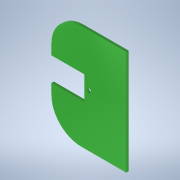
# Autodesk Inventor part: PCB-main
Saved by Autodesk Inventor 2022 (Build 260153000, 153)
## iProperties
Created: 2024-06-04
Part Number: PCB-main
Material: 一般
Document SubType Name: Modeling
Designer: yamashita1
Density: 1 g/cm^3
Appearance: 滑らか - 濃い深緑
Author: yamashita1
Autodesk Inventor part; units mm, degrees
ref_plane "YZ Plane" through (0, 0, 0) normal (1, 0, 0) x (0, 1, 0)
ref_plane "XZ Plane" through (0, 0, 0) normal (0, 1, 0) x (-1, 0, 0)
ref_plane "XY Plane" through (0, 0, 0) normal (0, 0, 1) x (1, 0, 0)
sketch "スケッチ1" plane through (0, 0, 0) normal (0, 0, 1) x (1, 0, 0)
  line L0 (-25, 35) -> (25, 35)
  line L1 (25, 35) -> (25, -35)
  line L2 (25, -35) -> (-25, -35)
  line L3 (-25, -35) -> (-25, 35)
  point P0 (0, 0)
  point P1 (-25, 0)
  point P2 (0, 35)
  dimension "d0" = 50
  dimension "d1" = 70
  constraints: 8 end point, 2 midpoint, 2 parallel, 1 horizontal, 1 horizontal alignment, 1 perpendicular, 1 vertical alignment
  measures "d0" distance of L1.end L2.end
  measures "d1" distance of L0.end L1.end
extrude "押し出し1" add sketch "スケッチ1" along normal blind 1.6
sketch "スケッチ2" plane through (0, 0, 1.6) normal (0, 0, 1) x (1, 0, 0)
  line L0 (-25, 35) -> (-25, -35) projected
  line L1 (-25, 8) -> (-3, 8)
  line L2 (-3, 8) -> (-3, -8)
  line L3 (-3, -8) -> (-25, -8)
  line L4 (-25, -8) -> (-25, 8)
  circle A0 centre (0, 0) radius 1.5
  point P0 (-25, 0)
  dimension "d10" = 16
  dimension "d11" = 3
  dimension "d12" = 25
  dimension "d13" = 3
  constraints: 8 end point, 2 midpoint, 2 parallel, 1 centre point, 1 coincident, 1 horizontal, 1 perpendicular, 1 point on line
  measures "d10" distance of L1.end L2.end
  measures "d11" diameter of A0
  measures "d12" distance from line of L0 A0.centre
  measures "d13" distance from line of L2 A0.centre
extrude "押し出し2" cut sketch "スケッチ2" against normal through all
fillet "フィレット1" radius 20 2 edges at (-25, -35, 0.8) (-25, 35, 0.8)
sketch "スケッチ3" plane through (0, 0, 1.6) normal (0, 0, 1) x (1, 0, 0)
  line L0 (25, -35) -> (25, 35) projected
  line L1 (25, 35) -> (-5, 35) projected
  line L2 (-30.9592, 0) -> (30.9592, 0) construction
  line L3 (-25, 8) -> (-3, 8) construction
  line L4 (-25, 15) -> (-25, 8) construction
  point P0 (0, 0)
  point P1 (-21, 12)
  point P2 (-21, -12)
  point P3 (21, -31)
  point P4 (21, 31)
  point P5 (0, 0)
  dimension "d15" = 4
  dimension "d16" = 4
  dimension "d17" = 4
  dimension "d18" = 4
  constraints: 2 end point, 2 symmetric about line, 1 coincident, 1 horizontal, 1 midpoint, 1 vertical alignment
  measures "d15" distance from line of L0 point (21, 31)
  measures "d16" distance from line of L1 point (21, 31)
  measures "d17" distance from line of L3 point (-21, 12)
  measures "d18" distance from line of L4 point (-21, 12)
hole "穴1" at (-21, 12, 1.6) at (-21, -12, 1.6) at (21, -31, 1.6) at (21, 31, 1.6) direction (0, 0, -1) diameter 3.2 end through all
equation "\"d16\" = d15"
equation "\"d17\" = d15"
equation "\"d18\" = d15"
